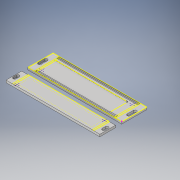
# Autodesk Inventor part: Button Fixture Base
Saved by Autodesk Inventor 2018 (Build 220112000, 112)
## iProperties
Created: 2016-07-07
Part Number: Button Fixture Base
Material: Generic
Document SubType Name: Modeling
Designer: Sam Clay
Density: 1 g/cm^3
Appearance: Default
Author: Sam Clay
Autodesk Inventor part; units mm, degrees
ref_plane "YZ Plane" through (0, 0, 0) normal (1, 0, 0) x (0, 1, 0)
ref_plane "XZ Plane" through (0, 0, 0) normal (0, 1, 0) x (-1, 0, 0)
ref_plane "XY Plane" through (0, 0, 0) normal (0, 0, 1) x (1, 0, 0)
sketch "Base Sketch" plane through (0, 0, 0) normal (0, 1, 0) x (-1, 0, 0)
  line L0 (0, 0) -> (660.4, 0)
  line L1 (660.4, 0) -> (660.4, 203.2)
  line L2 (660.4, 203.2) -> (0, 203.2)
  line L3 (0, 203.2) -> (0, 0)
  line L4 (660.4, 0) -> (711.2, 0)
  line L5 (711.2, 0) -> (711.2, 203.2)
  line L6 (711.2, 203.2) -> (660.4, 203.2)
  line L7 (660.4, 203.2) -> (660.4, 0)
  line L8 (0, 0) -> (-50.8, 0)
  line L9 (-50.8, 0) -> (-50.8, 203.2)
  line L10 (-50.8, 203.2) -> (0, 203.2)
  line L11 (0, 203.2) -> (0, 0)
  line L12 (711.2, 203.2) -> (-50.8, 203.2)
  line L13 (-50.8, 203.2) -> (-50.8, 254)
  line L14 (-50.8, 254) -> (711.2, 254)
  line L15 (711.2, 254) -> (711.2, 203.2)
  line L16 (-50.8, 254) -> (711.2, 254)
  line L17 (711.2, 254) -> (711.2, 381)
  line L18 (711.2, 381) -> (-50.8, 381)
  line L19 (-50.8, 381) -> (-50.8, 254)
  line L20 (660.4, 254) -> (660.4, 381)
  line L21 (0, 254) -> (0, 381)
  line L22 (647.7, 203.2) -> (647.7, 0)
  line L23 (12.7, 0) -> (12.7, 203.2)
  line L24 (12.7, 254) -> (12.7, 381)
  line L25 (647.7, 254) -> (647.7, 381)
  line L26 (628.65, 273.05) -> (31.75, 273.05) construction
  line L27 (31.75, 273.05) -> (31.75, 361.95) construction
  line L28 (31.75, 361.95) -> (628.65, 361.95) construction
  line L29 (628.65, 361.95) -> (628.65, 273.05) construction
  dimension "d0" = 660.4
  dimension "d1" = 203.2
  dimension "d2" = 50.8
  dimension "d3" = 50.8
  dimension "d79" = 50.8
  dimension "d80" = 127
  dimension "d81" = 12.7
  dimension "d82" = 12.7
  dimension "d83" = 50.8
  dimension "d84" = 50.8
  dimension "d85" = 19.05
  dimension "d86" = 19.05
  dimension "d87" = 19.05
  dimension "d88" = 19.05
  constraints: 60 end point, 19 point on line, 12 parallel, 10 perpendicular, 6 horizontal
  measures "d0" distance of L2.end L1.end
  measures "d1" distance of L1.end L0.end
  measures "d2" distance of L6.end L5.end
  measures "d3" distance of L9.end L10.end
  measures "d79" distance of L9.end L13.end
  measures "d80" distance of L17.end L16.end
  measures "d81" distance between parallel lines of L22 L1
  measures "d82" distance between parallel lines of L23 L3
  measures "d83" distance between parallel lines of L19 L21
  measures "d84" distance between parallel lines of L17 L20
  measures "d85" distance between parallel lines of L26 L14
  measures "d86" distance between parallel lines of L25 L29
  measures "d87" distance between parallel lines of L24 L27
  measures "d88" distance between parallel lines of L18 L28
extrude "Base" add sketch "Base Sketch" along normal blind 19.05 contours L3 L2 L23 L0 | L23 L2 L22 L0 | L22 L2 L1 L0 | L21 L18 L24 L14 | L24 L18 L25 L14 | L25 L18 L20 L14
extrude "Lower Level" add sketch "Base Sketch" along normal blind 17.78 contours L8 L9 L10 L3 | L1 L6 L5 L4 | L19 L18 L21 L14 | L14 L20 L18 L17
sketch "Track Sketch" plane through (0, 19.05, 0) normal (0, 1, 0) x (1, 0, 0)
  line L0 (0, 0) -> (-660.4, 0) projected
  line L1 (-660.4, 0) -> (-660.4, -203.2) projected
  line L2 (-660.4, -203.2) -> (0, -203.2) projected
  line L3 (0, -203.2) -> (0, 0) projected
  line L4 (-660.4, -3.175) -> (0, -3.175)
  line L5 (0, -203.2) -> (0, 0) projected
  line L6 (0, -22.987) -> (-660.4, -22.987)
  line L7 (-660.4, 0) -> (-660.4, -203.2) projected
  line L8 (-660.4, -200.025) -> (0, -200.025)
  line L9 (-660.4, -180.213) -> (0, -180.213)
  line L10 (-63.5, -40.767) -> (-660.4, -40.767)
  line L11 (-660.4, -40.767) -> (-660.4, -180.213)
  line L12 (-660.4, -180.213) -> (-63.5, -180.213)
  line L13 (-63.5, -180.213) -> (-63.5, -40.767)
  circle A0 centre (-68.58, -45.847) radius 8.89
  dimension "d91" = 3.175
  dimension "d92" = 19.812
  dimension "d93" = 17.78
  dimension "d94" = 63.5
  dimension "d95" = 3.175
  dimension "d96" = 19.812
  dimension "d97" = 17.78
  dimension "d98" = 5.08
  dimension "d99" = 5.08
  constraints: 16 end point, 8 point on line, 4 perpendicular, 2 horizontal, 2 parallel, 1 centre point
  measures "d91" distance between parallel lines of L4 L0
  measures "d92" distance between parallel lines of L6 L4
  measures "d93" distance between parallel lines of L6 L10
  measures "d94" distance between parallel lines of L3 L13
  measures "d95" distance between parallel lines of L2 L8
  measures "d96" distance between parallel lines of L12 L8
  measures "d97" diameter of A0
  measures "d98" distance from line of L13 A0.centre
  measures "d99" distance from line of A0.centre L10
extrude "Tracks Cut" cut sketch "Track Sketch" against normal blind 11.43 contours L3 L6 L1 L4 | L3 L8 L1 L9
extrude "Pocket Side" cut sketch "Track Sketch" against normal blind 3.175 contours L10 A0 L13 L9 L1 | A0 L13 L10 | L10 L13 A0
sketch "Origin Sketch" plane through (0, 19.05, 0) normal (0, 1, 0) x (1, 0, 0)
  line L0 (50.8, 0) -> (-711.2, 0) projected
  line L1 (50.8, -203.2) -> (50.8, 0) projected
  line L2 (-711.2, -203.2) -> (50.8, -203.2) projected
  line L3 (-711.2, 0) -> (-711.2, -203.2) projected
  line L4 (0, -203.2) -> (0, -200.025) projected
  line L5 (0, -203.2) -> (50.8, -203.2) projected
  line L6 (50.8, -203.2) -> (50.8, 0) projected
  line L7 (50.8, 0) -> (0, 0) projected
  line L8 (0, -3.175) -> (0, 0) projected
  line L9 (0, -22.987) -> (0, -3.175) projected
  line L10 (0, -180.213) -> (0, -22.987) projected
  line L11 (0, -200.025) -> (0, -180.213) projected
  line L12 (-660.4, -40.767) -> (-75.8756, -40.767) projected
  line L13 (0, -254) -> (-660.4, -254) projected
  line L14 (0, -381) -> (0, -254) projected
  line L15 (-628.65, -273.05) -> (-31.75, -273.05) construction
  line L16 (-628.65, -361.95) -> (-628.65, -273.05) construction
  line L17 (-31.75, -361.95) -> (-628.65, -361.95) construction
  line L18 (-31.75, -273.05) -> (-31.75, -361.95) construction
  line L19 (-12.7, -254) -> (-12.7, -381) projected
  line L20 (0, -254) -> (0, -381) projected
  line L21 (-660.4, -254) -> (-660.4, -381) projected
  line L22 (-647.7, -254) -> (-647.7, -381) projected
  line L23 (-647.7, -203.2) -> (-647.7, 0) projected
  line L24 (-660.4, 0) -> (-660.4, -203.2) projected
  line L25 (-12.7, 0) -> (-12.7, -203.2) projected
  line L26 (0, -203.2) -> (0, 0) projected
  line L27 (-63.5, -53.1426) -> (-63.5, -180.213) projected
  point P0 (-25.4, -40.767)
  point P1 (50.8, -203.2)
  point P2 (-635, -167.767)
  point P3 (-25.4, -266.7)
  point P4 (-635, -368.3)
  dimension "d72" = 127
  dimension "d73" = 609.6
  dimension "d100" = 25.4
  dimension "d102" = 12.7
  dimension "d103" = 25.4
  dimension "d127" = 101.6
  dimension "d128" = 609.6
  constraints: 1 point on line, 1 other
  measures "d72" vertical distance of point (-635, -167.767) point (-25.4, -40.767)
  measures "d73" horizontal distance of point (-635, -167.767) point (-25.4, -40.767)
  measures "d100" distance from line of L10 point (-25.4, -40.767)
  measures "d102" distance from line of point (-25.4, -266.7) L13
  measures "d103" distance from line of L14 point (-25.4, -266.7)
  measures "d127" vertical distance of point (-635, -368.3) point (-25.4, -266.7)
  measures "d128" horizontal distance of point (-635, -368.3) point (-25.4, -266.7)
sketch "Handles Sketch" plane through (0, 17.78, 0) normal (0, 1, 0) x (1, 0, 0)
  line L0 (-692.15, -63.5) -> (-692.15, -139.7) construction
  line L1 (-704.85, -76.2) -> (-704.85, -127)
  line L2 (-679.45, -127) -> (-679.45, -76.2)
  arc A0 (-679.45, -76.2) -> (-704.85, -76.2) centre (-692.15, -76.2) ccw
  arc A1 (-704.85, -127) -> (-679.45, -127) centre (-692.15, -127) ccw
  line L3 (-660.4, 0) -> (-711.2, 0) projected
  line L4 (-711.2, 0) -> (-711.2, -203.2) projected
  line L5 (50.8, -203.2) -> (50.8, 0) projected
  line L6 (-711.2, -203.2) -> (-660.4, -203.2) projected
  line L7 (-660.4, -254) -> (-711.2, -254) projected
  line L8 (-711.2, -381) -> (-660.4, -381) projected
  line L9 (-692.15, -292.1) -> (-692.15, -342.9) construction
  line L10 (-704.85, -304.8) -> (-704.85, -330.2)
  line L11 (-679.45, -330.2) -> (-679.45, -304.8)
  arc A2 (-679.45, -304.8) -> (-704.85, -304.8) centre (-692.15, -304.8) ccw
  arc A3 (-704.85, -330.2) -> (-679.45, -330.2) centre (-692.15, -330.2) ccw
  line L12 (31.75, -63.5) -> (31.75, -139.7) construction
  line L13 (19.05, -76.2) -> (19.05, -127)
  line L14 (44.45, -127) -> (44.45, -76.2)
  arc A4 (44.45, -76.2) -> (19.05, -76.2) centre (31.75, -76.2) ccw
  arc A5 (19.05, -127) -> (44.45, -127) centre (31.75, -127) ccw
  line L15 (31.75, -292.1) -> (31.75, -342.9) construction
  line L16 (19.05, -304.8) -> (19.05, -330.2)
  line L17 (44.45, -330.2) -> (44.45, -304.8)
  arc A6 (44.45, -304.8) -> (19.05, -304.8) centre (31.75, -304.8) ccw
  arc A7 (19.05, -330.2) -> (44.45, -330.2) centre (31.75, -330.2) ccw
  point P0 (0, 0)
  point P1 (31.75, -12.7)
  point P2 (31.75, -38.1)
  point P3 (31.75, -165.1)
  point P4 (31.75, -190.5)
  point P5 (31.75, -266.7)
  point P6 (31.75, -279.4)
  point P7 (31.75, -355.6)
  point P8 (31.75, -368.3)
  point P9 (-692.15, -368.3)
  point P10 (-692.15, -355.6)
  point P11 (-692.15, -279.4)
  point P12 (-692.15, -266.7)
  point P13 (-692.15, -190.5)
  point P14 (-692.15, -165.1)
  point P15 (-692.15, -38.1)
  point P16 (-692.15, -12.7)
  point P17 (-692.15, -101.6)
  point P18 (-692.15, -317.5)
  point P19 (31.75, -101.6)
  point P20 (31.75, -317.5)
  dimension "d104" = 76.2
  dimension "d105" = 25.4
  dimension "d106" = 101.6
  dimension "d107" = 19.05
  dimension "d108" = 19.05
  dimension "d109" = 19.05
  dimension "d110" = 12.7
  dimension "d111" = 25.4
  dimension "d112" = 12.7
  dimension "d113" = 25.4
  dimension "d114" = 12.7
  dimension "d115" = 12.7
  dimension "d116" = 12.7
  dimension "d117" = 12.7
  dimension "d118" = 50.8
  dimension "d119" = 25.4
  dimension "d120" = 63.5
  dimension "d121" = 76.2
  dimension "d122" = 25.4
  dimension "d123" = 50.8
  dimension "d124" = 25.4
  constraints: 32 end point, 24 point on circle, 17 vertical alignment, 16 tangent, 10 horizontal alignment, 10 point on line, 8 centre point, 4 midpoint, 4 parallel, 3 vertical
  measures "d104" distance of L0.start L0.end
  measures "d105" diameter of A1
  measures "d106" distance from line of point (-692.15, -101.6) L3
  measures "d107" distance from line of L4 point (-692.15, -101.6)
  measures "d108" distance from line of L4 point (-692.15, -12.7)
  measures "d109" distance from line of point (31.75, -12.7) L5
  measures "d110" distance from line of L3 point (-692.15, -12.7)
  measures "d111" distance of point (-692.15, -12.7) point (-692.15, -38.1)
  measures "d112" distance from line of L6 point (-692.15, -190.5)
  measures "d113" distance of point (-692.15, -165.1) point (-692.15, -190.5)
  measures "d114" distance from line of point (-692.15, -266.7) L7
  measures "d115" distance of point (-692.15, -266.7) point (-692.15, -279.4)
  measures "d116" distance from line of L8 point (-692.15, -368.3)
  measures "d117" distance of point (-692.15, -355.6) point (-692.15, -368.3)
  measures "d118" distance of L9.start L9.end
  measures "d119" diameter of A3
  measures "d120" distance from line of point (-692.15, -317.5) L7
  measures "d121" distance of L12.start L12.end
  measures "d122" diameter of A5
  measures "d123" distance of L15.start L15.end
  measures "d124" diameter of A7
extrude "Extrusion6" cut sketch "Handles Sketch" against normal through all
body "Solid1"
